robot-before-arms-2026-10-04 (Autodesk Fusion 360 design; units mm, degrees)
Autodesk Fusion 360 part; units mm, degrees
sketch "Layout_Side" plane through (0, 0, 0) normal (0, 1, 0) x (1, 0, 0) in component "00_Layout"
  line L0 (0, 0) -> (0, -1676.4) construction
  line L1 (300, -275) -> (-300, -275) construction
  line L2 (-300, -275) -> (-300, -75) construction
  line L3 (-300, -75) -> (300, -75) construction
  line L4 (300, -75) -> (300, -275) construction
  line L5 (300, -275) -> (-300, -75) construction
  line L6 (-300, -275) -> (300, -75) construction
  line L7 (0, -1676.4) -> (600, -1676.4) construction
  line L8 (0, -175) -> (0, -75) construction
  dimension "d1" = 200
  dimension "d2" = 600
  dimension "d4" = 600
  dimension "d5" = 75
  dimension "d6" = 1676.4
  constraint vertical L0
  constraint horizontal L1
  constraint perpendicular L1 L2
  constraint parallel L1 L3
  constraint parallel L2 L4
  constraint perpendicular L0 L7
  constraint midpoint L3 L8.end
  constraint coincident L0.start origin
  constraint midpoint L8.start L5
  measures "d1" distance of L1.end L2.end
  measures "d2" distance of L1.start L1.end
  measures "d4" distance of L0.end L7.end
  measures "d5" distance of L0.start L8.end
  measures "d6" distance of L0.end L0.start
sketch "Base_Profile" plane through (0, 0, 0) normal (0, 1, 0) x (1, 0, 0) in component "01_Base_Envelope"
  line L0 (300, -275) -> (-300, -275)
  line L1 (-300, -275) -> (-300, -75)
  line L2 (-300, -75) -> (300, -75)
  line L3 (300, -75) -> (300, -275)
extrude "Chassis_Width_450mm" add sketch "Base_Profile" along normal mid plane 450 makes body 1 in component "01_Base_Envelope"
sketch "Mast_Envelope_Side_Profile" plane through (0, 0, 0) normal (0, 1, 0) x (1, 0, 0) in component "02_Mast_Envelope"
  line L0 (-160, -275) -> (-40, -275)
  line L1 (-40, -275) -> (-40, -1600)
  line L2 (-40, -1600) -> (-160, -1600)
  line L3 (-160, -1600) -> (-160, -275)
  line L4 (300, -275) -> (-300, -275) construction
  dimension "d9" = 120
  dimension "d10" = 1325
  dimension "d11" = 160
  constraint horizontal L0
  constraint vertical L1
  constraint horizontal L2
  constraint vertical L3
  constraint coincident L0.start L4
  measures "d9" horizontal distance of L0.start L0.end
  measures "d10" vertical distance of L0.end L1.end
  measures "d11" horizontal distance of origin L0.start
extrude "Mast_Envelope_Width_140mm" add sketch "Mast_Envelope_Side_Profile" along normal mid plane 140 separate body makes body 2 in component "02_Mast_Envelope"
sketch "Shared_Carriage_Side_Profile" plane through (0, 0, 0) normal (0, 1, 0) x (1, 0, 0) in component "03_Shared_Carriage"
  line L0 (-40, -840) -> (80, -840)
  line L1 (80, -840) -> (80, -960)
  line L2 (80, -960) -> (-40, -960)
  line L3 (-40, -960) -> (-40, -840)
  dimension "d14" = 120
  dimension "d15" = 120
  dimension "d16" = 40
  dimension "d17" = 840
  constraint horizontal L0
  constraint vertical L1
  constraint horizontal L2
  constraint vertical L3
  measures "d14" horizontal distance of L0.start L0.end
  measures "d15" vertical distance of L0.end L1.end
  measures "d16" horizontal distance of origin L0.start
  measures "d17" vertical distance of origin L0.start
extrude "Shared_Carriage_Width_660mm" add sketch "Shared_Carriage_Side_Profile" along normal mid plane 660 separate body makes body 3 in component "03_Shared_Carriage"
ref_plane "WorkPlane1" through (0, 300, 0) normal (0, 1, 0) x (0, 0, 1) in component "00_Layout"
sketch "Reach_Left_Floor_2x304p8mm" plane through (0, 300, 0) normal (0, 1, 0) x (1, 0, 0) in component "00_Layout"
  circle A0 centre (80, -400) radius 609.6 construction
  line L0 (80, -400) -> (380.0994, -346.6765) construction
  line L1 (380.0994, -346.6765) -> (450, -50) construction
  dimension "d25" = 80
  dimension "d26" = 400
  dimension "d27" = 450
  dimension "d28" = 50
  dimension "d29" = 609.6
  dimension "d30" = 304.8
  dimension "d31" = 304.8
  measures "d25" horizontal distance of origin A0.centre
  measures "d26" vertical distance of origin A0.centre
  measures "d27" horizontal distance of origin L1.end
  measures "d28" vertical distance of origin L1.end
  measures "d29" radius of A0
  measures "d30" distance of A0.centre L0.end
  measures "d31" distance of L1.end L0.end
sketch "Reach_Left_Shelf_2x304p8mm" plane through (0, 300, 0) normal (0, 1, 0) x (1, 0, 0) in component "00_Layout"
  circle A0 centre (80, -1400) radius 609.6 construction
  line L0 (80, -1400) -> (198.6357, -1680.7643) construction
  line L1 (198.6357, -1680.7643) -> (500, -1726.4) construction
  dimension "d32" = 80
  dimension "d33" = 1400
  dimension "d34" = 500
  dimension "d35" = 1726.4
  dimension "d36" = 609.6
  dimension "d37" = 304.8
  dimension "d38" = 304.8
  measures "d32" horizontal distance of origin A0.centre
  measures "d33" vertical distance of origin A0.centre
  measures "d34" horizontal distance of origin L1.end
  measures "d35" vertical distance of origin L1.end
  measures "d36" radius of A0
  measures "d37" distance of A0.centre L0.end
  measures "d38" distance of L1.end L0.end
ref_plane "WorkPlane2" through (0, -300, 0) normal (0, 1, 0) x (0, 0, 1) in component "00_Layout"
sketch "Reach_Right_Floor_2x304p8mm" plane through (0, -300, 0) normal (0, 1, 0) x (1, 0, 0) in component "00_Layout"
  circle A0 centre (80, -400) radius 609.6 construction
  line L0 (80, -400) -> (380.0994, -346.6765) construction
  line L1 (380.0994, -346.6765) -> (450, -50) construction
  dimension "d41" = 80
  dimension "d42" = 400
  dimension "d43" = 450
  dimension "d44" = 50
  dimension "d45" = 609.6
  dimension "d46" = 304.8
  dimension "d47" = 304.8
  measures "d41" horizontal distance of origin A0.centre
  measures "d42" vertical distance of origin A0.centre
  measures "d43" horizontal distance of origin L1.end
  measures "d44" vertical distance of origin L1.end
  measures "d45" radius of A0
  measures "d46" distance of A0.centre L0.end
  measures "d47" distance of L1.end L0.end
sketch "Reach_Right_Shelf_2x304p8mm" plane through (0, -300, 0) normal (0, 1, 0) x (1, 0, 0) in component "00_Layout"
  circle A0 centre (80, -1400) radius 609.6 construction
  line L0 (80, -1400) -> (198.6357, -1680.7643) construction
  line L1 (198.6357, -1680.7643) -> (500, -1726.4) construction
  dimension "d48" = 80
  dimension "d49" = 1400
  dimension "d50" = 500
  dimension "d51" = 1726.4
  dimension "d52" = 609.6
  dimension "d53" = 304.8
  dimension "d54" = 304.8
  measures "d48" horizontal distance of origin A0.centre
  measures "d49" vertical distance of origin A0.centre
  measures "d50" horizontal distance of origin L1.end
  measures "d51" vertical distance of origin L1.end
  measures "d52" radius of A0
  measures "d53" distance of A0.centre L0.end
  measures "d54" distance of L1.end L0.end
component "00_Layout" placed x (1, 0, 0) y (0, 1, 0) z (0, 0, 1) at (0, 0, 0)
component "01_Base_Envelope" placed x (1, 0, 0) y (0, 1, 0) z (0, 0, 1) at (0, 0, 0)
component "02_Mast_Envelope" placed x (1, 0, 0) y (0, 1, 0) z (0, 0, 1) at (0, 0, 0)
component "03_Shared_Carriage" placed x (1, 0, 0) y (0, 1, 0) z (0, 0, 1) at (0, 0, 0)
named bodies: "Chassis_Envelope", "Mast_Envelope_Packaging_Only", "Shared_Carriage_Packaging_Only"
